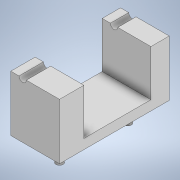
# Autodesk Inventor part: Support_2B
Saved by Autodesk Inventor 2021 (Build 250183000, 183)
## iProperties
Created: 2021-04-14
Part Number: Support_2B
Material: Generic
Document SubType Name: Modeling
Designer: Jawal
Density: 1 g/cm^3
Appearance: Default
Author: Jawal
Autodesk Inventor part; units mm, degrees
ref_plane "YZ Plane" through (0, 0, 0) normal (1, 0, 0) x (0, 1, 0)
ref_plane "XZ Plane" through (0, 0, 0) normal (0, 1, 0) x (-1, 0, 0)
ref_plane "XY Plane" through (0, 0, 0) normal (0, 0, 1) x (1, 0, 0)
sketch "Sketch1" plane through (0, 0, 0) normal (1, 0, 0) x (0, 1, 0)
  line L0 (11.4385, 17.5) -> (-11.4385, 17.5)
  line L1 (-11.4385, 17.5) -> (-11.4385, -27.5)
  line L2 (-11.4385, -27.5) -> (11.4385, -27.5)
  line L3 (11.4385, -27.5) -> (11.4385, 17.5)
  point P0 (0, 0)
  dimension "d0" = 45
  dimension "d1" = 22.877
  dimension "d2" = 11.4385
  dimension "d15" = 17.5
  constraints: 8 end point, 2 parallel, 1 horizontal, 1 perpendicular
  measures "d0" distance of L2.end L0.start
  measures "d1" distance of L1.end L2.end
  measures "d2" distance from line of point (0, 0) L3
  measures "d15" distance from line of L0 point (0, 0)
extrude "Extrusion1" add sketch "Sketch1" along normal blind 20
sketch "Sketch2" plane through (0, -11.4385, -27.5) normal (0, -1, 0) x (1, 0, 0)
  circle A0 centre (16.5, 41.5) radius 1.5
  circle A1 centre (16.5, 13.5) radius 1.5
  line L0 (0, 0) -> (20, 0) projected
  line L1 (0, 45) -> (20, 45) projected
  line L2 (20, 0) -> (20, 45) projected
  point P0 (0, 27.5)
  dimension "d6" = 3
  dimension "d7" = 3
  dimension "d8" = 28
  dimension "d10" = 3.5
  dimension "d12" = 3.5
  constraints: 2 centre point
  measures "d6" diameter of A0
  measures "d7" diameter of A1
  measures "d8" distance of A1.centre A0.centre
  measures "d10" distance from line of L1 A0.centre
  measures "d12" distance from line of L2 A0.centre
extrude "Extrusion2" add sketch "Sketch2" along normal blind 3
sketch "Sketch3" plane through (20, 0, 0) normal (1, 0, 0) x (0, 0, -1)
  line L0 (27.5, 11.4385) -> (-17.5, 11.4385) projected
  line L1 (-7.5, 11.4385) -> (20, 11.4385)
  line L2 (20, 11.4385) -> (20, -7.4385)
  line L3 (20, -7.4385) -> (-7.5, -7.4385)
  line L4 (-7.5, -7.4385) -> (-7.5, 11.4385)
  line L5 (27.5, -11.4385) -> (27.5, 11.4385) projected
  line L6 (-17.5, -11.4385) -> (27.5, -11.4385) projected
  line L7 (-17.5, 11.4385) -> (-17.5, -11.4385) projected
  point P0 (0, 0)
  dimension "d17" = 7.5
  dimension "d18" = 4
  dimension "d25" = 10
  constraints: 8 end point, 2 parallel, 1 horizontal, 1 perpendicular, 1 point on line
  measures "d17" distance between parallel lines of L2 L5
  measures "d18" distance between parallel lines of L6 L3
  measures "d25" distance between parallel lines of L7 L4
extrude "Extrusion3" cut sketch "Sketch3" against normal through all contours L2 L3 L4 L0
sketch "Sketch4" plane through (0, -11.4385, -27.5) normal (0, 0, -1) x (-1, 0, 0)
  line L0 (0, 22.877) -> (-20, 22.877) projected
  arc A0 (-6.387, 22.877) -> (-3.387, 22.877) centre (-4.887, 22.877) ccw
  line L1 (-20, 0) -> (-20, 22.877) projected
  point P0 (0, 11.4385)
  dimension "d21" = 3
  dimension "d22" = 15.113
  constraints: 3 point on line, 2 point on circle, 1 centre point
  measures "d21" diameter of A0
  measures "d22" distance from line of L1 A0.centre
extrude "Extrusion4" cut sketch "Sketch4" against normal through all
equation "\"d2\" = 0.5 * d1"
body "Solid1"
